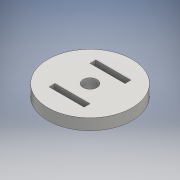
# Autodesk Inventor part: leva00
Saved by Autodesk Inventor 2016 (Build 200138000, 138)
## iProperties
Created: 2016-09-20
Part Number: leva00
Material: Madera (abedul)
Document SubType Name: Modeling
Designer: i95sa
Density: 0.55 g/cm^3
Appearance: Suave - Blanco
Author: i95sa
Autodesk Inventor part; units mm, degrees
ref_plane "YZ Plane" through (0, 0, 0) normal (1, 0, 0) x (0, 1, 0)
ref_plane "XZ Plane" through (0, 0, 0) normal (0, 1, 0) x (-1, 0, 0)
ref_plane "XY Plane" through (0, 0, 0) normal (0, 0, 1) x (1, 0, 0)
sketch "Boceto1" plane through (0, 0, 0) normal (0, 0, 1) x (1, 0, 0)
  arc A0 (30, 0) -> (-30, 0) centre (0, 0) ccw
  line L0 (5, 0) -> (30, 0)
  arc A1 (-30, 0) -> (30, 0) centre (0, 0) ccw
  circle A2 centre (0, 0) radius 5
  line L1 (0, 0) -> (0, 12.5)
  line L2 (0, 12.5) -> (-12.5, 12.5)
  line L3 (-12.5, 12.5) -> (-12.5, 16.7)
  line L4 (-12.5, 16.7) -> (12.5, 16.7)
  line L5 (12.5, 16.7) -> (12.5, 12.5)
  line L6 (12.5, 12.5) -> (0, 12.5)
  line L7 (0, 0) -> (0, -12.5)
  line L8 (0, -12.5) -> (-12.5, -12.5)
  line L9 (-12.5, -12.5) -> (-12.5, -16.7)
  line L10 (-12.5, -16.7) -> (12.5, -16.7)
  line L11 (12.5, -16.7) -> (12.5, -12.5)
  line L12 (0, -12.5) -> (12.5, -12.5)
  point P0 (0.3554, 29.9979)
  point P1 (0.3554, -29.9979)
  point P2 (-5, 0)
  dimension "d0" = 60
  dimension "d13" = 10
  dimension "d14" = 12.5
  dimension "d15" = 12.5
  dimension "d16" = 4.2
  dimension "d17" = 25
  dimension "d18" = 12.5
  dimension "d19" = 12.5
  dimension "d20" = 4.2
  dimension "d21" = 25
  constraints: 26 end point, 8 point on circle, 7 point on line, 5 perpendicular, 3 centre point, 3 coincident, 1 horizontal, 1 parallel, 1 vertical
  measures "d0" diameter of A0
  measures "d13" diameter of A2
  measures "d14" distance of L1.start L1.end
  measures "d15" distance of L1.end L2.end
  measures "d16" distance of L2.end L3.end
  measures "d17" distance of L3.end L4.end
  measures "d18" distance of L1.start L7.end
  measures "d19" distance of L7.end L8.end
  measures "d20" distance of L8.end L9.end
  measures "d21" distance of L9.end L10.end
extrude "Extrusión2" add sketch "Boceto1" along normal blind 8
